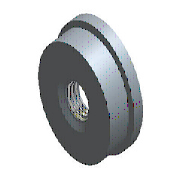
# Autodesk Inventor part: PR10-M5
Saved by Autodesk Inventor 2021.1 (Build 251245000, 245)
## iProperties
IsCustomPart: 1
Created: 2020-01-21
Part Number: PR10-M5
Material: Stainless Steel
Catalog Web Link: www.pemnet.com
Description: PEM Brand Access Hardware PR10 - Metric
Vendor: PennEngineering®
Document SubType Name: Modeling
Standard: PEM
Designer: alid
Manufacturer: PennEngineering®
Language: en-US
Size Designation: PR10-M5
Categories: <MemberInstance><Categories><Category DisplayName="Sheet Metal" InternalName="21944ee9-ad4d-44c9-9b1e-873eb7935d2a" Mnemonic="PEM"><Category DisplayName="Nuts" InternalName="15e34f97-5541-421a-a775-44d98c1adcde" Mnemonic="pemNut"><CategoryParameter DisplayName="Nominal Diameter" InternalName="0be71e27-5492-4f5f-b057-e8c8d33d0305" Mnemonic="nomdia"/><CategoryParameter DisplayName="Thread Class" InternalName="2354338d-f827-46bd-8778-0ed3d7286146" Mnemonic="thrclss"/><CategoryParameter DisplayName="Thread Series Designation" InternalName="571a622b-fa51-4821-aeeb-e24f544f017e" Mnemonic="thrserdsgn"/><CategoryParameter DisplayName="Hole diameter" InternalName="5cda2139-ecc7-4f59-8502-3162f0124b70" Mnemonic="SMNHD"/><CategoryParameter DisplayName="Threads per Unit" InternalName="64655984-9347-4d07-8751-37792c28ecd8" Mnemonic="thrperunit1"/><CategoryParameter DisplayName="Thread Type" InternalName="7a3892cf-1811-453a-b9c2-22c8b70c36bf" Mnemonic="thrtype"/><CategoryParameter DisplayName="Thread Length" InternalName="a5235de7-e741-4b6b-b2e9-a6829ffd9d3f" Mnemonic="thrlen"/><CategoryParameter DisplayName="Thread Designation" InternalName="ab33a7e4-2ca9-400b-8e2d-5973b7f77f2c" Mnemonic="thrdesign"/><CategoryParameter DisplayName="Height" InternalName="c013d27b-95cd-4187-8e83-a1be557daece" Mnemonic="nheig"/><CategoryParameter DisplayName="Min sheet thickness" InternalName="ff2eaae3-31bc-42d2-bfe3-2e39a04c80e9" Mnemonic="SMNMIST"/></Category></Category><Category DisplayName="DataType" InternalName="23b78d0f-2648-40c6-8793-ca6db495c9e8" Mnemonic="DATATYPE"><CategoryParameter DisplayName="DisplayName" InternalName="05415f3d-3907-474b-a020-eb9d644f4cf3" Mnemonic="DISPLAYNAME"/><CategoryParameter DisplayName="Standard" InternalName="0c0a119c-1e12-4c84-803f-101930972f5e" Mnemonic="STANDARD"/><CategoryParameter DisplayName="Description" InternalName="13903e3d-64b1-4950-80da-f627842ea37f" Mnemonic="DESCRIPTION"/><CategoryParameter DisplayName="Designation" InternalName="2675968c-4ce5-49e0-a4f5-552d29089031" Mnemonic="DESIGNATION"/><CategoryParameter DisplayName="Default Row" InternalName="2af9ec52-faaa-4026-b378-f9fa4afca842" Mnemonic="DEFAULTROW"/><CategoryParameter DisplayName="Folder Name" InternalName="3f06958e-8713-4116-9be7-ed6184ecc97b" Mnemonic="FOLDERNAME"/><CategoryParameter DisplayName="Revision Guid" InternalName="45a75005-10b1-4dfc-8d6d-dfe629f0b93c" Mnemonic="REVISIONGUID"/><CategoryParameter DisplayName="FileName" InternalName="8b46a4cc-9585-4fed-90c3-899f57e09a73" Mnemonic="FILENAME"/><CategoryParameter DisplayName="StdsOrg" InternalName="8f5914e1-4693-403f-8ab5-d37768198c9d" Mnemonic="STDSORG"/><CategoryParameter DisplayName="Family Version" InternalName="914462f6-6e19-4b14-ba84-155b9680b1d0" Mnemonic="FAMILYREVISION"/><CategoryParameter DisplayName="Standard Revision" InternalName="91d5a463-65c2-4fde-b823-3b7fea5e8e17" Mnemonic="STANDARDREVISION"/><CategoryParameter DisplayName="Member Revision" InternalName="a65d44b9-392f-4f4f-857b-e4b3d54996fe" Mnemonic="MEMBERREVISION"/><CategoryParameter DisplayName="ClipFormat" InternalName="bc51e27b-3422-4e78-93ef-cec197ddf230" Mnemonic="CLIPFORMAT"/><CategoryParameter DisplayName="Manufacturer" InternalName="cd6c7a72-a28a-4e50-99a9-2c7f4e13e5ad" Mnemonic="MANUFACTURER"/><CategoryParameter DisplayName="InternalName" InternalName="cf1d0246-76d9-4b4a-8305-fa0409afb5c1" Mnemonic="INTERNALNAME"/><CategoryParameter DisplayName="IsMetric" InternalName="e2385c5b-1ea4-4823-96a8-8de651266ec3" Mnemonic="ISMETRIC"/><Category DisplayName="Part" InternalName="c0e0b642-3bcb-4cc8-9e80-f96d35c4afa4" Mnemonic="PART"><CategoryParameter DisplayName="Part Number" InternalName="016b6077-bfbe-49bd-92c9-d8d59c39c941" Mnemonic="PARTNUMBER"/><CategoryParameter DisplayName="Stock Number" InternalName="4dba7c1c-e26c-444e-836c-b08b433409a8" Mnemonic="STOCKNUMBER"/><CategoryParameter DisplayName="Material Key" InternalName="5c9a8adb-dd2b-4535-b97f-0a94a95fe41f" Mnemonic="MATERIALKEY"/><CategoryParameter DisplayName="Material" InternalName="818a152a-d3c3-49ca-80ee-df7d91421b8e" Mnemonic="MATERIAL"/></Category></Category></Categories><FamilyTemplate Id="PEM Brand Access Hardware PR10 - Metric"><FamilyTemplateParameters><FamilyTemplateParameter ObjectType="kUserParameterObject" ValueType="xs:double" Id="1" ObjectReferenceKey="A_"/><FamilyTemplateParameter ObjectType="kUserParameterObject" ValueType="xs:double" Id="2" ObjectReferenceKey="B"/><FamilyTemplateParameter ObjectType="kUserParameterObject" ValueType="xs:double" Id="3" ObjectReferenceKey="C_"/><FamilyTemplateParameter ObjectType="kUserParameterObject" ValueType="xs:double" Id="4" ObjectReferenceKey="E_"/><FamilyTemplateParameter ObjectType="kUserParameterObject" ValueType="xs:double" Id="9" ObjectReferenceKey="H_"/><FamilyTemplateParameter ObjectType="kUserParameterObject" ValueType="xs:double" Id="10" ObjectReferenceKey="H_Size"/><FamilyTemplateParameter ObjectType="kUserParameterObject" ValueType="xs:double" Id="11" ObjectReferenceKey="Min_Dist"/><FamilyTemplateParameter ObjectType="kUserParameterObject" ValueType="xs:double" Id="12" ObjectReferenceKey="Min_Sheet_for_Flush_Installation"/><FamilyTemplateParameter ObjectType="kUserParameterObject" ValueType="xs:double" Id="13" ObjectReferenceKey="Min_Sheet_for_Self_Clinching"/><FamilyTemplateParameter ObjectType="kUserParameterObject" ValueType="xs:double" Id="14" ObjectReferenceKey="NND"/><FamilyTemplateParameter ObjectType="kUserParameterObject" ValueType="xs:double" Id="16" ObjectReferenceKey="TD_d"/><FamilyTemplateParameter ObjectType="kUserParameterObject" ValueType="xs:double" Id="17" ObjectReferenceKey="TL"/><FamilyTemplateParameter ObjectType="kPropertyObject" ValueType="xs:string" Id="100" ObjectReferenceKey="{32853F0F-3444-11d1-9E93-0060B03C1CA6}" SubObjectId="52"/><FamilyTemplateParameter ObjectType="kPropertyObject" ValueType="xs:string" Id="105" ObjectReferenceKey="{32853F0F-3444-11d1-9E93-0060B03C1CA6}" SubObjectId="5"/><FamilyTemplateParameter ObjectType="kPartComponentDefinitionObject" ValueType="xs:string" Id="110" SubObjectId="Material"/><FamilyTemplateParameter ObjectType="kThreadFeatureObject" ValueType="xs:structure" Id="300" ObjectReferenceKey="1002000010000000d61c0000000000008000000000000000" SubObjectId="ThreadInfo"><FamilyTemplateParameter ObjectType="" ValueType="xs:string" Id="301" SubObjectId="ThreadClass"/><FamilyTemplateParameter ObjectType="" ValueType="xs:string" Id="302" SubObjectId="ThreadDesignation"/><FamilyTemplateParameter ObjectType="" ValueType="xs:string" Id="303" SubObjectId="ThreadType"/><FamilyTemplateParameter ObjectType="" ValueType="xs:string" Id="304" SubObjectId="Pitch"/><FamilyTemplateParameter ObjectType="" ValueType="xs:string" Id="305" SubObjectId="ThreadType"/></FamilyTemplateParameter></FamilyTemplateParameters></FamilyTemplate><CategoryParameterMap><ParamToTemplateMap><ParamToTemplate CategoryParameter="//CategoryParameter[@InternalName='7a3892cf-1811-453a-b9c2-22c8b70c36bf']" ConstantValue=""/><ParamToTemplate CategoryParameter="//CategoryParameter[@InternalName='05415f3d-3907-474b-a020-eb9d644f4cf3']" ConstantValue="PEM Brand Access Hardware PR10 - Metric"/><ParamToTemplate CategoryParameter="//CategoryParameter[@InternalName='0c0a119c-1e12-4c84-803f-101930972f5e']" ConstantValue="PEM"/><ParamToTemplate CategoryParameter="//CategoryParameter[@InternalName='13903e3d-64b1-4950-80da-f627842ea37f']" ConstantValue="PEM Brand Access Hardware PR10 - Metric"/><ParamToTemplate CategoryParameter="//CategoryParameter[@InternalName='2af9ec52-faaa-4026-b378-f9fa4afca842']" ConstantValue="1"/><ParamToTemplate CategoryParameter="//CategoryParameter[@InternalName='3f06958e-8713-4116-9be7-ed6184ecc97b']" ConstantValue="PEM Brand Access Hardware PR10 - Metric"/><ParamToTemplate CategoryParameter="//CategoryParameter[@InternalName='45a75005-10b1-4dfc-8d6d-dfe629f0b93c']" ConstantValue="7e12bf44-08d1-42c2-b907-b96c0fc436a5"/><ParamToTemplate CategoryParameter="//CategoryParameter[@InternalName='8f5914e1-4693-403f-8ab5-d37768198c9d']" TemplateParameter="101"/><ParamToTemplate CategoryParameter="//CategoryParameter[@InternalName='914462f6-6e19-4b14-ba84-155b9680b1d0']" ConstantValue="11"/><ParamToTemplate CategoryParameter="//CategoryParameter[@InternalName='91d5a463-65c2-4fde-b823-3b7fea5e8e17']" TemplateParameter="103"/><ParamToTemplate CategoryParameter="//CategoryParameter[@InternalName='bc51e27b-3422-4e78-93ef-cec197ddf230']" ConstantValue="CF_INVENTOR.STDPARTS"/><ParamToTemplate CategoryParameter="//CategoryParameter[@InternalName='cd6c7a72-a28a-4e50-99a9-2c7f4e13e5ad']" ConstantValue="PennEngineering®"/><ParamToTemplate CategoryParameter="//CategoryParameter[@InternalName='cf1d0246-76d9-4b4a-8305-fa0409afb5c1']" ConstantValue="c7157d83-91f8-4fb1-9d47-9d41ee379006"/><ParamToTemplate CategoryParameter="//CategoryParameter[@InternalName='e2385c5b-1ea4-4823-96a8-8de651266ec3']" ConstantValue="true"/><ParamToTemplate CategoryParameter="//CategoryParameter[@InternalName='8b46a4cc-9585-4fed-90c3-899f57e09a73']" ConstantValue="PR10-M5"/><ParamToTemplate CategoryParameter="//CategoryParameter[@InternalName='a65d44b9-392f-4f4f-857b-e4b3d54996fe']" ConstantValue="e6920fca-6b60-4445-9ffb-76a34294bd9f"/><ParamToTemplate CategoryParameter="//CategoryParameter[@InternalName='c013d27b-95cd-4187-8e83-a1be557daece']" TemplateParameter="1"/><ParamToTemplate CategoryParameter="//CategoryParameter[@InternalName='2675968c-4ce5-49e0-a4f5-552d29089031']" TemplateParameter="100"/><ParamToTemplate CategoryParameter="//CategoryParameter[@InternalName='5cda2139-ecc7-4f59-8502-3162f0124b70']" TemplateParameter="10"/><ParamToTemplate CategoryParameter="//CategoryParameter[@InternalName='2354338d-f827-46bd-8778-0ed3d7286146']" TemplateParameter="301"/><ParamToTemplate CategoryParameter="//CategoryParameter[@InternalName='ab33a7e4-2ca9-400b-8e2d-5973b7f77f2c']" TemplateParameter="302"/><ParamToTemplate CategoryParameter="//CategoryParameter[@InternalName='818a152a-d3c3-49ca-80ee-df7d91421b8e']" TemplateParameter="110"/><ParamToTemplate CategoryParameter="//CategoryParameter[@InternalName='ff2eaae3-31bc-42d2-bfe3-2e39a04c80e9']" TemplateParameter="12"/><ParamToTemplate CategoryParameter="//CategoryParameter[@InternalName='0be71e27-5492-4f5f-b057-e8c8d33d0305']" TemplateParameter="14"/><ParamToTemplate CategoryParameter="//CategoryParameter[@InternalName='016b6077-bfbe-49bd-92c9-d8d59c39c941']" TemplateParameter="105"/><ParamToTemplate CategoryParameter="//CategoryParameter[@InternalName='a5235de7-e741-4b6b-b2e9-a6829ffd9d3f']" TemplateParameter="17"/></ParamToTemplateMap></CategoryParameterMap></MemberInstance>
Density: 8 g/cm^3
Appearance: Semi-Polished
Title: Retainer
Author: alid
Revision Number: A
Autodesk Inventor part; units mm, degrees
ref_plane "YZ Plane" through (0, 0, 0) normal (1, 0, 0) x (0, 1, 0)
ref_plane "XZ Plane" through (0, 0, 0) normal (0, 1, 0) x (-1, 0, 0)
ref_plane "XY Plane" through (0, 0, 0) normal (0, 0, 1) x (1, 0, 0)
sketch "Sketch1" plane through (0, 0, 0) normal (1, 0, 0) x (0, 1, 0)
  line L0 (0, 0) -> (4.75, 0)
  line L1 (4.75, 0) -> (4.75, 2.025)
  line L2 (4.75, 2.025) -> (4.55, 2.025)
  line L3 (4.55, 2.025) -> (4.55, 2.225)
  line L4 (4.55, 2.225) -> (5.205, 2.225)
  line L5 (5.205, 2.225) -> (5.205, 3.18)
  line L6 (5.205, 3.18) -> (3.885, 3.18)
  line L7 (3.685, 2.98) -> (3.685, 1.27)
  line L8 (3.685, 1.27) -> (0, 1.27)
  line L9 (0, 1.27) -> (0, 0)
  line L10 (3.885, 3.18) -> (3.685, 2.98)
  point P0 (3.685, 3.18)
  dimension "d1" = 9.5
  dimension "d4" = 0.2
  dimension "d5" = 3.18
  dimension "d6" = 10.41
  dimension "d7" = 1.91
  dimension "d8" = 7.37
  dimension "d9" = 0.955
  dimension "d28" = 0.2
  dimension "d29" = 0.2
  constraints: 22 end point, 8 parallel, 2 perpendicular, 2 point on line, 1 horizontal
  measures "d1" diameter of L1 L9
  measures "d4" distance of L2.end L3.end
  measures "d5" distance between parallel lines of L0 L6
  measures "d6" diameter of L5 L9
  measures "d7" distance between parallel lines of L6 L8
  measures "d8" diameter of L7 L9
  measures "d9" distance of L4.end L5.end
  measures "d28" distance of L6.end point (3.685, 3.18)
  measures "d29" distance of L7.start point (3.685, 3.18)
revolve "Revolution1" add sketch "Sketch1" angle 360 about axis through (0, 0, 1.27) along (0, 0, -1)
hole "Hole1" at (0, 0, 0) direction (0, 0, 1) diameter 4.134 end through all countersink diameter 5.25 countersink angle 120 thread size "M5x0.8" class "6H" standard "ANSI Metric M Profile"
equation "\"d1\" = C_"
equation "\"d4\" = TD_d"
equation "\"d5\" = A_"
equation "\"d6\" = E_"
equation "\"d7\" = H_"
equation "\"d8\" = B"
equation "\"d9\" = 0.5 * H_"
equation "\"d28\" = TD_d"
equation "\"d29\" = d28"
equation "\"d19\" = 1.05 * NND"
equation "\"A_\" = 3.18"
equation "\"B\" = 7.37"
equation "\"C_\" = 9.5"
equation "\"E_\" = 10.41"
equation "\"H_\" = 1.91"
equation "\"NND\" = 5"
equation "\"TD_d\" = 0.2"
equation "\"Min_Sheet_for_Self_Clinching\" = 1.27"
equation "\"Min_Sheet_for_Flush_Installation\" = 3.18"
equation "\"Min_Dist\" = 9.14"
equation "\"H_Size\" = 9.53"
equation "\"TL\" = 1.27"
body "Solid1"
